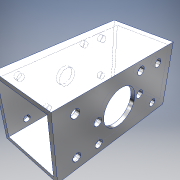
# Autodesk Inventor part: Arm 4 inch
Saved by Autodesk Inventor 2019 (Build 230136000, 136)
## iProperties
Created: 2018-09-22
Part Number: Arm 4 inch
Material: Aluminum 6061
Document SubType Name: Modeling
Designer: Adhik
Density: 2.7 g/cm^3
Appearance: Aluminum - Flat
Mass: 155.95 g
Surface Area: 388.179 cm^2
Volume: 57.7592 cm^3
Author: Adhik
Autodesk Inventor part; units mm, degrees
ref_plane "YZ Plane" through (0, 0, 0) normal (1, 0, 0) x (0, 1, 0)
ref_plane "XZ Plane" through (0, 0, 0) normal (0, 1, 0) x (-1, 0, 0)
ref_plane "XY Plane" through (0, 0, 0) normal (0, 0, 1) x (1, 0, 0)
sketch "Sketch1" plane through (0, 0, 0) normal (0, 0, 1) x (1, 0, 0)
  line L0 (-35.56, 0) -> (35.56, 0) construction
  line L1 (0, -35.56) -> (0, 35.56) construction
  line L2 (-25.4, 25.4) -> (25.4, 25.4)
  line L3 (25.4, 25.4) -> (25.4, -25.4)
  line L4 (25.4, -25.4) -> (-25.4, -25.4)
  line L5 (-25.4, -25.4) -> (-25.4, 25.4)
  line L6 (-22.225, 22.225) -> (22.225, 22.225)
  line L7 (22.225, 22.225) -> (22.225, -22.225)
  line L8 (22.225, -22.225) -> (-22.225, -22.225)
  line L9 (-22.225, -22.225) -> (-22.225, 22.225)
  point P0 (0, 0)
  point P1 (-25.4, 0)
  point P2 (0, 25.4)
  point P3 (-22.225, 0)
  point P4 (0, 22.225)
  dimension "d0" = 50.8
  dimension "d1" = 3.175
  dimension "d11" = 50.8
  dimension "d12" = 3.175
  constraints: 16 end point, 4 midpoint, 4 parallel, 4 point on line, 2 horizontal, 2 perpendicular
  measures "d0" distance of L4.end L2.start
  measures "d1" distance between parallel lines of L2 L6
  measures "d11" distance of L2.start L2.end
  measures "d12" distance between parallel lines of L5 L9
extrude "Extrusion1" add sketch "Sketch1" along normal mid plane 101.6
sketch "Sketch6" plane through (-25.4, -25.4, 50.8) normal (-1, 0, 0) x (0, 0, 1)
  circle A0 centre (-68.7605, 43.3605) radius 2.0193 construction
  circle A1 centre (-32.8395, 7.4395) radius 2.0193 construction
  circle A2 centre (-50.8, 25.4) radius 6.985 projected
  line L0 (0, 47.625) -> (-101.6, 47.625) construction
  line L1 (-101.6, 3.175) -> (-101.6, 47.625) construction
  line L2 (0, 3.175) -> (-101.6, 3.175) construction
  line L3 (0, 47.625) -> (0, 3.175) construction
  circle A3 centre (-86.7029, 41.275) radius 3.175 projected
  circle A4 centre (-14.8971, 9.525) radius 3.175 projected
  circle A5 centre (-86.7029, 9.525) radius 3.175 projected
  circle A6 centre (-14.8971, 41.275) radius 3.175 projected
  circle A7 centre (-68.7605, 43.3605) radius 2.413
  circle A8 centre (-32.8395, 7.4395) radius 2.413
  point P0 (-50.8, 25.4)
  dimension "d38" = 4.826
  constraints: 2 centre point, 2 coincident, 1 equal radius
  measures "d38" diameter of A7
sketch "Sketch7" plane through (25.4, -25.4, 50.8) normal (1, 0, 0) x (0, 0, -1)
  circle A0 centre (50.8, 25.4) radius 14.2875
  dimension "d25" = 28.575
  constraints: 1 centre point, 1 coincident
  measures "d25" diameter of A0
extrude "Extrusion8" cut sketch "Sketch7" against normal up to next
sketch "Sketch8" plane through (-22.225, -22.225, -50.8) normal (1, 0, 0) x (0, 0, -1)
  circle A0 centre (-14.8971, 6.35) radius 2.667 projected
  circle A1 centre (-86.7029, 6.35) radius 2.667 projected
  circle A2 centre (-86.7029, 38.1) radius 2.667 projected
  circle A3 centre (-14.8971, 38.1) radius 2.667 projected
  point P0 (-50.8, 22.225)
extrude "Extrusion9" cut sketch "Sketch8" against normal up to next
sketch "Sketch9" plane through (25.4, -25.4, 50.8) normal (1, 0, 0) x (0, 0, -1)
  circle A0 centre (14.8971, 9.525) radius 3.175 projected
  circle A1 centre (14.8971, 41.275) radius 3.175 projected
  circle A2 centre (86.7029, 9.525) radius 3.175 projected
  circle A3 centre (86.7029, 41.275) radius 3.175 projected
  point P0 (50.8, 25.4)
extrude "Extrusion10" cut sketch "Sketch9" against normal up to next
sketch "Sketch10" plane through (22.225, -22.225, -50.8) normal (-1, 0, 0) x (0, 0, 1)
  circle A0 centre (69.85, 22.225) radius 2.667 construction
  circle A1 centre (31.75, 22.225) radius 2.667 construction
  circle A2 centre (69.85, 22.225) radius 3.175
  circle A3 centre (31.75, 22.225) radius 3.175
  point P0 (50.8, 22.225)
  dimension "d32" = 6.35
  constraints: 2 centre point, 2 coincident, 1 equal radius
  measures "d32" diameter of A2
extrude "Extrusion11" cut sketch "Sketch10" against normal through all
sketch "Sketch11" plane through (25.4, -25.4, 50.8) normal (1, 0, 0) x (0, 0, -1)
  circle A0 centre (68.7605, 43.3605) radius 2.0193 construction
  circle A1 centre (32.8395, 7.4395) radius 2.0193 construction
  circle A2 centre (68.7605, 43.3605) radius 3.175
  circle A3 centre (32.8395, 7.4395) radius 3.175
  point P0 (50.8, 25.4)
  dimension "d35" = 6.35
  constraints: 2 centre point, 2 coincident, 1 equal radius
  measures "d35" diameter of A3
extrude "Extrusion12" cut sketch "Sketch11" against normal up to next
extrude "Extrusion13" cut sketch "Sketch6" against normal up to next contours A2 | A7 | A8
equation "\"d12\" = d1"
body "Solid1"
